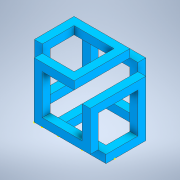
# Autodesk Inventor part: WeirdCube
Saved by Autodesk Inventor 2020.1 (Build 241239000, 239)
## iProperties
Created: 2019-09-30
Part Number: WeirdCube
Material: Generic
Document SubType Name: Modeling
Designer: super
Density: 1 g/cm^3
Appearance: Default
Author: super
Autodesk Inventor part; units mm, degrees
ref_plane "YZ Plane" through (0, 0, 0) normal (1, 0, 0) x (0, 1, 0)
ref_plane "XZ Plane" through (0, 0, 0) normal (0, 1, 0) x (-1, 0, 0)
ref_plane "XY Plane" through (0, 0, 0) normal (0, 0, 1) x (1, 0, 0)
sketch "Sketch1" plane through (0, 0, 0) normal (0, 1, 0) x (-1, 0, 0)
  line L0 (0, 0) -> (0, -70)
  line L1 (0, -70) -> (70, -70)
  line L2 (70, -70) -> (70, 0)
  line L3 (70, 0) -> (0, 0)
  dimension "d0" = 70
  dimension "d1" = 70
  dimension "d2" = 70
  constraints: 8 end point, 2 perpendicular, 1 vertical
  measures "d0" distance of L0.start L0.end
  measures "d1" distance of L0.end L1.end
  measures "d2" distance of L1.end L2.end
extrude "Extrusion1" add sketch "Sketch1" along normal blind 10
sketch "Sketch2" plane through (0, 10, 0) normal (0, 1, 0) x (1, 0, 0)
  line L0 (-10, 10) -> (-10, 60)
  line L1 (-10, 60) -> (-60, 60)
  line L2 (-60, 60) -> (-60, 10)
  line L3 (-60, 10) -> (-10, 10)
  point P0 (0, 0)
  dimension "d7" = 50
  dimension "d8" = 50
  dimension "d9" = 50
  constraints: 8 end point, 2 perpendicular, 1 horizontal
  measures "d7" distance of L0.start L0.end
  measures "d8" distance of L0.end L1.end
  measures "d9" distance of L1.end L2.end
extrude "Extrusion2" cut sketch "Sketch2" against normal blind 10
sketch "Sketch3" plane through (0, 10, 0) normal (0, 1, 0) x (1, 0, 0)
  line L0 (0, 70) -> (-70, 70) projected
  line L1 (0, 70) -> (0, 60)
  line L2 (0, 0) -> (0, 70) projected
  line L3 (0, 60) -> (-10, 60)
  line L4 (-10, 60) -> (-10, 70)
  dimension "d12" = 10
  dimension "d13" = 10
  dimension "d14" = 10
  constraints: 6 end point, 1 perpendicular, 1 point on line
  measures "d12" distance of L0.start L1.end
  measures "d13" distance of L1.end L3.end
  measures "d14" distance of L3.end L4.end
extrude "Extrusion3" cut sketch "Sketch3" against normal blind 10
sketch "Sketch4" plane through (0, 10, 0) normal (0, 1, 0) x (1, 0, 0)
  line L0 (-10, 60) -> (-60, 60) projected
  line L1 (-10, 60) -> (-10, 50)
  line L2 (-10, 60) -> (-10, 10) projected
  line L3 (-10, 50) -> (0, 50)
  line L4 (0, 0) -> (0, 60) projected
  line L5 (0, 50) -> (0, 60)
  line L6 (-10, 60) -> (0, 60) projected
  line L7 (0, 60) -> (-10, 60)
  dimension "d17" = 10
  dimension "d18" = 10
  dimension "d19" = 10
  dimension "d20" = 10
  constraints: 8 end point, 2 point on line, 1 collinear, 1 perpendicular
  measures "d17" distance of L0.start L1.end
  measures "d18" distance of L1.end L3.end
  measures "d19" distance of L3.end L4.end
  measures "d20" distance of L4.end L0.start
extrude "Extrusion4" cut sketch "Sketch4" against normal blind 10
sketch "Sketch5" plane through (0, 10, 0) normal (0, 1, 0) x (1, 0, 0)
  line L0 (-10, 60) -> (-10, 70) projected
  line L1 (-10, 60) -> (-10, 70)
  line L2 (-10, 70) -> (-20, 70)
  line L3 (-10, 70) -> (-70, 70) projected
  line L4 (-20, 70) -> (-20, 60)
  line L5 (-60, 60) -> (-10, 60) projected
  line L6 (-20, 60) -> (-10, 60)
  point P0 (0, 0)
  dimension "d23" = 10
  dimension "d24" = 10
  dimension "d25" = 10
  dimension "d26" = 10
  constraints: 8 end point, 1 collinear, 1 perpendicular, 1 point on line
  measures "d23" distance of L0.start L0.end
  measures "d24" distance of L0.end L2.end
  measures "d25" distance of L2.end L4.end
  measures "d26" distance of L4.end L0.start
extrude "Extrusion5" cut sketch "Sketch5" against normal blind 10
sketch "Sketch6" plane through (0, 10, 0) normal (0, 1, 0) x (1, 0, 0)
  line L0 (-10, 50) -> (0, 50) projected
  line L1 (-10, 50) -> (-10, 40)
  line L2 (-10, 40) -> (0, 40)
  line L3 (0, 0) -> (0, 50) projected
  line L4 (0, 40) -> (0, 50)
  line L5 (0, 50) -> (-10, 50)
  dimension "d29" = 10
  dimension "d30" = 10
  dimension "d31" = 10
  dimension "d32" = 10
  constraints: 8 end point, 1 collinear, 1 perpendicular, 1 point on line, 1 vertical
  measures "d29" distance of L0.start L1.end
  measures "d30" distance of L1.end L2.end
  measures "d31" distance of L2.end L0.end
  measures "d32" distance of L0.end L0.start
extrude "Extrusion6" add sketch "Sketch6" along normal blind 70
sketch "Sketch7" plane through (0, 10, 0) normal (0, 1, 0) x (1, 0, 0)
  line L0 (-20, 60) -> (-30, 60)
  line L1 (-60, 60) -> (-20, 60) projected
  line L2 (-30, 60) -> (-30, 70)
  line L3 (-20, 70) -> (-70, 70) projected
  line L4 (-30, 70) -> (-20, 70)
  line L5 (-20, 70) -> (-20, 60)
  point P0 (0, 0)
  dimension "d35" = 10
  dimension "d36" = 10
  dimension "d37" = 10
  dimension "d38" = 10
  constraints: 8 end point, 2 point on line, 1 collinear, 1 perpendicular
  measures "d35" distance of L0.start L0.end
  measures "d36" distance of L0.end L2.end
  measures "d37" distance of L2.end L3.start
  measures "d38" distance of L3.start L0.start
extrude "Extrusion7" add sketch "Sketch7" along normal blind 60
sketch "Sketch8" plane through (0, 80, 0) normal (0, 1, 0) x (1, 0, 0)
  line L0 (0, 40) -> (-10, 40) projected
  line L1 (0, 40) -> (0, 50)
  line L2 (-10, 50) -> (0, 50) projected
  line L3 (0, 50) -> (-10, 50)
  line L4 (-10, 50) -> (-10, 40)
  line L5 (-10, 40) -> (0, 40)
  point P0 (0, 0)
  dimension "d41" = 10
  dimension "d42" = 10
  dimension "d43" = 10
  dimension "d44" = 10
  constraints: 8 end point, 1 collinear, 1 perpendicular, 1 vertical
  measures "d41" distance of L0.start L1.end
  measures "d42" distance of L1.end L2.start
  measures "d43" distance of L2.start L4.end
  measures "d44" distance of L4.end L0.start
extrude "Extrusion8" cut sketch "Sketch8" against normal blind 10
sketch "Sketch9" plane through (-10, 10, -40) normal (0, 0, 1) x (1, 0, 0)
  line L0 (10, 60) -> (0, 60) projected
  line L1 (0, 60) -> (0, 50)
  line L2 (0, 60) -> (0, -10) projected
  line L3 (0, 50) -> (10, 50)
  line L4 (10, -10) -> (10, 60) projected
  line L5 (10, 50) -> (10, 60)
  line L6 (10, 60) -> (0, 60)
  dimension "d47" = 10
  dimension "d48" = 10
  dimension "d49" = 10
  dimension "d50" = 10
  constraints: 8 end point, 2 point on line, 1 perpendicular
  measures "d47" distance of L0.end L1.end
  measures "d48" distance of L1.end L3.end
  measures "d49" distance of L3.end L0.start
  measures "d50" distance of L0.start L0.end
extrude "Extrusion9" add sketch "Sketch9" along normal blind 60
sketch "Sketch10" plane through (-10, 60, -40) normal (0, -1, 0) x (1, 0, 0)
  line L0 (10, 60) -> (0, 60) projected
  line L1 (0, 60) -> (10, 60)
  line L2 (10, 60) -> (10, 50)
  line L3 (10, -10) -> (10, 60) projected
  line L4 (10, 50) -> (0, 50)
  line L5 (0, 60) -> (0, -10) projected
  line L6 (0, 50) -> (0, 60)
  point P0 (10, 40)
  dimension "d53" = 10
  dimension "d54" = 10
  dimension "d55" = 10
  dimension "d56" = 10
  constraints: 8 end point, 2 collinear, 2 point on line
  measures "d53" distance of L0.end L0.start
  measures "d54" distance of L0.start L2.end
  measures "d55" distance of L2.end L4.end
  measures "d56" distance of L4.end L0.end
extrude "Extrusion10" add sketch "Sketch10" along normal blind 40
sketch "Sketch11" plane through (-10, 0, -10) normal (-1, 0, 0) x (0, 0, 1)
  line L0 (20, 20) -> (30, 20) projected
  line L1 (20, 20) -> (30, 20)
  line L2 (30, 20) -> (30, 30)
  line L3 (30, 70) -> (30, 20) projected
  line L4 (30, 30) -> (20, 30)
  line L5 (20, 60) -> (20, 20) projected
  line L6 (20, 30) -> (20, 20)
  point P0 (10, 0)
  dimension "d59" = 10
  dimension "d60" = 10
  dimension "d61" = 10
  dimension "d62" = 10
  constraints: 8 end point, 2 point on line, 1 collinear
  measures "d59" distance of L0.start L0.end
  measures "d60" distance of L0.end L2.end
  measures "d61" distance of L2.end L4.end
  measures "d62" distance of L4.end L0.start
extrude "Extrusion11" add sketch "Sketch11" along normal blind 50
sketch "Sketch12" plane through (-30, 10, -70) normal (-1, 0, 0) x (0, 0, 1)
  line L0 (0, 60) -> (0, -10) projected
  line L1 (10, 60) -> (0, 60) projected
  line L2 (0, 60) -> (10, 60)
  line L3 (10, 60) -> (10, 50)
  line L4 (10, -10) -> (10, 60) projected
  line L5 (10, 50) -> (0, 50)
  line L6 (0, 50) -> (0, 60)
  line L7 (0, 60) -> (0, 55)
  point P0 (70, -10)
  dimension "d65" = 10
  dimension "d66" = 10
  dimension "d67" = 10
  dimension "d68" = 10
  constraints: 10 end point, 2 point on line, 1 collinear, 1 horizontal, 1 midpoint
  measures "d65" distance of L0.start L1.start
  measures "d66" distance of L1.start L3.end
  measures "d67" distance of L3.end L5.end
  measures "d68" distance of L5.end L0.start
extrude "Extrusion12" add sketch "Sketch12" along normal blind 60
sketch "Sketch13" plane through (-90, 10, -70) normal (-1, 0, 0) x (0, 0, 1)
  point P0 (70, -10)
sketch "Sketch14" plane through (-30, 60, -70) normal (0, -1, 0) x (1, 0, 0)
  line L0 (10, 0) -> (-60, 0) projected
  line L1 (-60, 0) -> (-60, 10) projected
  line L2 (-60, 0) -> (-60, 10)
  line L3 (-60, 10) -> (-50, 10)
  line L4 (10, 10) -> (-60, 10) projected
  line L5 (-50, 10) -> (-50, 0)
  line L6 (-50, 0) -> (-60, 0)
  point P0 (30, 70)
  dimension "d71" = 10
  dimension "d72" = 10
  dimension "d73" = 10
  dimension "d74" = 10
  constraints: 8 end point, 1 perpendicular, 1 point on line, 1 vertical
  measures "d71" distance of L0.end L1.end
  measures "d72" distance of L1.end L3.end
  measures "d73" distance of L3.end L5.end
  measures "d74" distance of L5.end L0.end
extrude "Extrusion13" add sketch "Sketch14" along normal blind 40
sketch "Sketch15" plane through (-60, 0, -60) normal (0, 0, 1) x (1, 0, 0)
  line L0 (-20, 20) -> (-30, 20) projected
  line L1 (-30, 20) -> (-20, 20)
  line L2 (-20, 20) -> (-20, 30)
  line L3 (-20, 60) -> (-20, 20) projected
  line L4 (-20, 30) -> (-30, 30)
  line L5 (-30, 70) -> (-30, 20) projected
  line L6 (-30, 30) -> (-30, 20)
  point P0 (60, 0)
  dimension "d77" = 10
  dimension "d78" = 10
  dimension "d79" = 10
  dimension "d80" = 10
  constraints: 8 end point, 2 point on line, 1 collinear
  measures "d77" distance of L0.end L0.start
  measures "d78" distance of L0.start L2.end
  measures "d79" distance of L2.end L4.end
  measures "d80" distance of L4.end L0.end
extrude "Extrusion14" add sketch "Sketch15" along normal blind 60
sketch "Sketch16" plane through (-60, 0, -10) normal (-1, 0, 0) x (0, 0, 1)
  point P0 (10, 0)
sketch "Sketch17" plane through (-60, 0, -10) normal (-1, 0, 0) x (0, 0, 1)
  line L0 (20, 20) -> (30, 20) projected
  line L1 (30, 20) -> (20, 20)
  line L2 (20, 20) -> (20, 30)
  line L3 (20, 60) -> (20, 20) projected
  line L4 (20, 30) -> (30, 30)
  line L5 (30, 70) -> (30, 20) projected
  line L6 (30, 30) -> (30, 20)
  point P0 (10, 0)
  dimension "d83" = 10
  dimension "d84" = 10
  dimension "d85" = 10
  dimension "d86" = 10
  constraints: 8 end point, 1 collinear, 1 perpendicular, 1 point on line
  measures "d83" distance of L0.end L0.start
  measures "d84" distance of L0.start L2.end
  measures "d85" distance of L2.end L4.end
  measures "d86" distance of L4.end L0.end
extrude "Extrusion15" add sketch "Sketch17" along normal blind 10
sketch "Sketch18" plane through (-90, 30, -60) normal (0, 1, 0) x (1, 0, 0)
  line L0 (90, -70) -> (20, -70) projected
  line L1 (20, -70) -> (20, -80)
  line L2 (20, -80) -> (30, -80)
  line L3 (30, -80) -> (30, -70)
  line L4 (30, -70) -> (20, -70)
  point P0 (90, -60)
  dimension "d89" = 10
  dimension "d90" = 10
  dimension "d91" = 10
  dimension "d92" = 10
  constraints: 8 end point, 1 collinear, 1 perpendicular, 1 point on line, 1 vertical
  measures "d89" distance of L0.end L1.end
  measures "d90" distance of L1.end L2.end
  measures "d91" distance of L2.end L3.end
  measures "d92" distance of L3.end L0.end
extrude "Extrusion16" add sketch "Sketch18" along normal blind 60
sketch "Sketch19" plane through (-60, 30, 10) normal (1, 0, 0) x (0, 0, -1)
  line L0 (-10, 60) -> (0, 60)
  line L1 (0, 60) -> (0, 50)
  line L2 (0, 50) -> (-10, 50)
  line L3 (-10, 0) -> (-10, 60) projected
  line L4 (-10, 50) -> (-10, 60)
  point P0 (10, -30)
  dimension "d95" = 10
  dimension "d96" = 10
  dimension "d97" = 10
  dimension "d98" = 10
  constraints: 8 end point, 2 perpendicular, 1 horizontal
  measures "d95" distance of L0.start L0.end
  measures "d96" distance of L0.end L1.end
  measures "d97" distance of L1.end L2.end
  measures "d98" distance of L2.end L0.start
extrude "Extrusion17" add sketch "Sketch19" along normal blind 40
sketch "Sketch20" plane through (-90, 30, -60) normal (0, 1, 0) x (1, 0, 0)
  line L0 (0.0426, -60) -> (0, -50.0001)
  line L1 (0, 0) -> (0, -60) projected
  line L2 (0, -50.0001) -> (9.9999, -49.9575)
  line L3 (9.9999, -49.9575) -> (10.0425, -59.9574)
  line L4 (10.0425, -59.9574) -> (0.0426, -60)
  point P0 (90, -60)
  dimension "d101" = 10
  dimension "d102" = 10
  dimension "d103" = 10
  dimension "d104" = 10
  constraints: 8 end point, 2 perpendicular, 1 point on line
  measures "d101" distance of L0.start L0.end
  measures "d102" distance of L0.end L2.end
  measures "d103" distance of L2.end L3.end
  measures "d104" distance of L3.end L0.start
extrude "Extrusion18" add sketch "Sketch20" along normal blind 60
sketch "Sketch21" plane through (-90, 30, -9.9999) normal (-0.0042561, 0, -0.9999909) x (-0.9999909, 0, 0.0042561)
  point P0 (-89.9566, -30)
sketch "Sketch22" plane through (-90, 30, -9.9999) normal (-0.0042561, 0, -0.9999909) x (-0.9999909, 0, 0.0042561)
  line L0 (0, 60) -> (-10, 60) projected
  line L1 (-10, 60) -> (0, 60)
  line L2 (0, 60) -> (0, 50)
  line L3 (0, 0) -> (0, 60) projected
  line L4 (0, 50) -> (-10, 50)
  line L5 (-10, 0) -> (-10, 60) projected
  line L6 (-10, 50) -> (-10, 60)
  point P0 (-89.9566, -30)
  dimension "d107" = 10
  dimension "d108" = 10
  dimension "d109" = 10
  dimension "d110" = 10
  constraints: 8 end point, 2 collinear, 2 point on line
  measures "d107" distance of L0.end L0.start
  measures "d108" distance of L0.start L2.end
  measures "d109" distance of L2.end L4.end
  measures "d110" distance of L4.end L0.end
extrude "Extrusion19" add sketch "Sketch22" along normal blind 40
sketch "Sketch23" plane through (0, 60, 10) normal (0, 0, -1) x (-1, 0, 0)
  line L0 (70, 30) -> (20, 30) projected
  line L1 (20, 20) -> (20, 30) projected
  line L2 (20, 30) -> (20, 20)
  line L3 (20, 20) -> (30, 20)
  line L4 (60, 20) -> (20, 20) projected
  line L5 (30, 20) -> (30, 30)
  line L6 (30, 30) -> (20, 30)
  point P0 (0, -60)
  dimension "d113" = 10
  dimension "d114" = 10
  dimension "d115" = 10
  dimension "d116" = 10
  constraints: 8 end point, 2 point on line, 1 vertical
  measures "d113" distance of L0.end L1.start
  measures "d114" distance of L1.start L3.end
  measures "d115" distance of L3.end L5.end
  measures "d116" distance of L5.end L0.end
extrude "Extrusion20" add sketch "Sketch23" along normal blind 60
sketch "Sketch24" plane through (-79.9575, 30, -0.0426) normal (0.9999909, 0, -0.0042561) x (-0.0042561, 0, -0.9999909)
  point P0 (-0.3829, -30)
sketch "Sketch25" plane through (-30, 80, 10) normal (-1, 0, 0) x (0, 0, 1)
  point P0 (-10, -80)
sketch "Sketch26" plane through (-30, 80, 10) normal (-1, 0, 0) x (0, 0, 1)
  line L0 (0, 10) -> (-60, 10) projected
  line L1 (-60, 10) -> (-60, 0)
  line L2 (-60, 0) -> (-50, 0)
  line L3 (0, 0) -> (-60, 0) projected
  line L4 (-50, 0) -> (-50, 10)
  line L5 (-50, 10) -> (-60, 10)
  point P0 (-10, -80)
  dimension "d119" = 10
  dimension "d120" = 10
  dimension "d121" = 10
  dimension "d122" = 10
  constraints: 8 end point, 1 perpendicular, 1 point on line, 1 vertical
  measures "d119" distance of L0.end L1.end
  measures "d120" distance of L1.end L2.end
  measures "d121" distance of L2.end L4.end
  measures "d122" distance of L4.end L0.end
extrude "Extrusion21" add sketch "Sketch26" along normal blind 60
body "Solid1"
